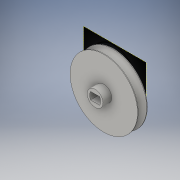
# Autodesk Inventor part: Wheel
Saved by Autodesk Inventor 2016 (Build 200138000, 138)
## iProperties
Created: 2017-09-08
Part Number: Wheel
Material: Generic
Document SubType Name: Modeling
Designer: student
Density: 1 g/cm^3
Appearance: Default
Author: student
Autodesk Inventor part; units mm, degrees
ref_plane "YZ Plane" through (0, 0, 0) normal (1, 0, 0) x (0, 1, 0)
ref_plane "XZ Plane" through (0, 0, 0) normal (0, 1, 0) x (-1, 0, 0)
sketch "Sketch1" plane through (0, 0, 0) normal (0, 0, 1) x (1, 0, 0)
  circle A0 centre (0, 0) radius 21.717
  dimension "d0" = 43.434
  constraints: 1 centre point, 1 coincident
  measures "d0" diameter of A0
extrude "Extrusion1" add sketch "Sketch1" along normal blind 6.35
sketch "Sketch2" plane through (0, 0, 0) normal (1, 0, 0) x (0, 1, 0)
  line L0 (-21.717, 0) -> (-21.717, 6.35) projected
  circle A0 centre (-21.717, 3.175) radius 2.7305
  point P0 (0, 0)
  dimension "d3" = 5.461
  constraints: 1 centre point, 1 midpoint
  measures "d3" diameter of A0
ref_plane "Work Plane1" through (0, 0, 3.175) normal (0, 0, 1) x (1, 0, 0)
sketch "Sketch3" plane through (0, 0, 3.175) normal (0, 0, 1) x (1, 0, 0)
  circle A0 centre (0, 0) radius 21.717
  dimension "d4" = 43.434
  constraints: 1 centre point, 1 coincident
  measures "d4" diameter of A0
sweep "Sweep1" cut profiles "Sketch2" path "Sketch3"
sketch "Sketch4" plane through (0, 0, 6.35) normal (0, 0, 1) x (1, 0, 0)
  circle A0 centre (0, 0) radius 5.08
  line L0 (3.4671, -2.3876) -> (-3.4671, -2.3876)
  line L1 (-3.4671, -2.3876) -> (-3.4671, 2.3876)
  line L2 (-3.4671, 2.3876) -> (3.4671, 2.3876)
  line L3 (3.4671, 2.3876) -> (3.4671, -2.3876)
  line L4 (3.4671, -2.3876) -> (-3.4671, 2.3876) construction
  line L5 (-3.4671, -2.3876) -> (3.4671, 2.3876) construction
  dimension "d7" = 10.16
  dimension "d8" = 6.9342
  dimension "d9" = 4.7752
  constraints: 12 end point, 2 midpoint, 2 parallel, 1 centre point, 1 coincident, 1 horizontal, 1 perpendicular
  measures "d7" diameter of A0
  measures "d8" distance of L1.end L2.end
  measures "d9" distance of L0.end L1.end
extrude "Extrusion2" add sketch "Sketch4" along normal blind 5.588 contours A0 | L0 L1 L2 L3
sketch "Sketch6" plane through (0, 0, 11.938) normal (0, 0, 1) x (1, 0, 0)
  line L0 (2.9579, -2.3876) -> (-2.9579, -2.3876)
  line L1 (-2.9579, 2.3876) -> (2.9579, 2.3876)
  arc A0 (-2.9579, 2.3876) -> (-2.9579, -2.3876) centre (2.3852, 0) ccw
  arc A1 (2.9579, -2.3876) -> (2.9579, 2.3876) centre (-2.3852, 0) ccw
  constraints: 4 end point, 4 point on circle, 2 centre point, 1 horizontal, 1 parallel
extrude "Extrusion4" cut sketch "Sketch6" against normal blind 5.588
sketch "Sketch7" plane through (0, 0, 0) normal (0, 0, -1) x (-1, 0, 0)
  line L0 (-20.8863, 24.5767) -> (19.4, 24.5767) construction
  line L1 (19.4, 24.5767) -> (19.4, -5.9629) construction
  line L2 (19.4, -5.9629) -> (-20.8863, -5.9629) construction
  line L3 (-20.8863, -5.9629) -> (-20.8863, 24.5767) construction
  line L4 (0, -0.3242) -> (-9.8884, 9.9119)
  line L5 (-9.8884, 9.9119) -> (-7.7165, 12.5279)
  line L6 (-7.7165, 12.5279) -> (-2.5005, 8.5874)
  line L7 (0, -0.3242) -> (9.8165, 10.0936)
  line L8 (9.8165, 10.0936) -> (7.8287, 12.3794)
  line L9 (7.8287, 12.3794) -> (2.5792, 8.5874)
  line L10 (-2.5005, 8.5874) -> (-1.0716, 11.9114)
  arc A0 (0.5712, 12.9625) -> (-1.0716, 11.9114) centre (0.3003, 11.5765) ccw
  arc A1 (2.807, 12.2818) -> (0.5712, 12.9625) centre (0.8004, 9.7033) ccw
  line L11 (2.807, 12.2818) -> (2.807, 11.5765)
  arc A2 (2.807, 11.5765) -> (1.5855, 10.7693) centre (2.2208, 11.1357) ccw
  line L12 (1.5855, 10.7693) -> (2.5792, 8.5874)
  circle A3 centre (0, 0) radius 5.08 projected
  constraints: 18 end point, 6 point on circle, 3 centre point, 1 vertical, 2 other
body "Solid1"
